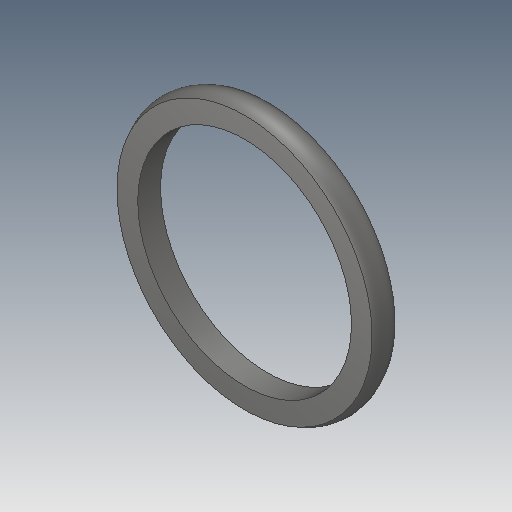
# Autodesk Inventor part: OIL RING
Saved by Autodesk Inventor 2019 (Build 230136000, 136)
## iProperties
Created: 2023-06-18
Part Number: OIL RING
Material: Generic
Document SubType Name: Modeling
Designer: Fransic
Density: 1 g/cm^3
Appearance: Rubber - Black - Version 1.1
Mass: 3.57268 g
Surface Area: 28.4752 cm^2
Volume: 3.57268 cm^3
Author: Fransic
Autodesk Inventor part; units mm, degrees
ref_plane "YZ Plane" through (0, 0, 0) normal (1, 0, 0) x (0, 1, 0)
ref_plane "XZ Plane" through (0, 0, 0) normal (0, 1, 0) x (-1, 0, 0)
ref_plane "XY Plane" through (0, 0, 0) normal (0, 0, 1) x (1, 0, 0)
sketch "Sketch1" plane through (0, 0, 0) normal (0, 1, 0) x (-1, 0, 0)
  line L0 (22.1944, 0) -> (26.5, 0)
  line L1 (26.5, 0) -> (26.5, -4.7394)
  line L2 (26.5, -4.7394) -> (22.1944, -4.7394)
  line L3 (0, -4.7394) -> (0, 0)
  line L4 (22.1944, 0) -> (22.1944, -4.7394)
  arc A0 (26.5, -4.7394) -> (26.5, 0) centre (23.5178, -2.3697) ccw
  dimension "d0" = 26.5
  constraints: 10 end point, 2 parallel, 2 perpendicular, 2 point on circle, 1 centre point, 1 horizontal
  measures "d0" distance of L1.end L3.start
revolve "Revolution1" add sketch "Sketch1" angle 360 about axis through (0, 0, -4.7394) along (0, 0, 1)
body "Solid1"
